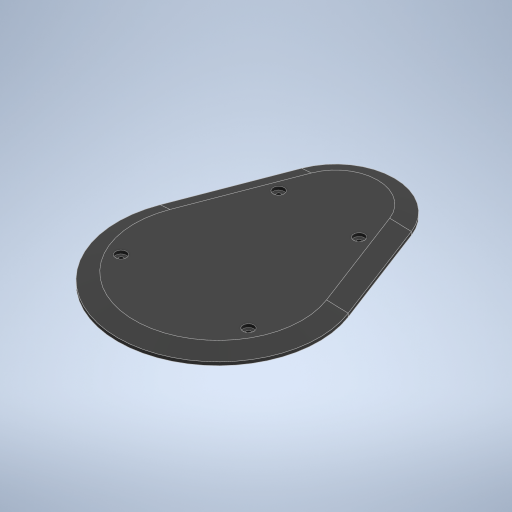
# Autodesk Inventor part: Arm_1_Cover
Saved by Autodesk Inventor 2023 (Build 270158000, 158)
## iProperties
Created: 2024-07-29
Part Number: Arm_1_Cover
Material: Generic
Document SubType Name: Modeling
Designer: Swoby
Density: 1 g/cm^3
Appearance: Default
Author: Swoby
Autodesk Inventor part; units mm, degrees
ref_plane "YZ Plane" through (0, 0, 0) normal (1, 0, 0) x (0, 1, 0)
ref_plane "XZ Plane" through (0, 0, 0) normal (0, 1, 0) x (-1, 0, 0)
ref_plane "XY Plane" through (0, 0, 0) normal (0, 0, 1) x (1, 0, 0)
sketch "Sketch1" plane through (0, 0, 0) normal (0, 1, 0) x (-1, 0, 0)
  arc A0 (28.0215, -10.7143) -> (-28.0215, -10.7143) centre (0, 0) ccw
  arc A1 (14.9976, -25.9821) -> (-16.3459, -41.25) centre (0, -35) ccw construction
  line L0 (0, 0) -> (0, -35) construction
  line L1 (-28.0215, -10.7143) -> (-16.3459, -41.25)
  line L2 (16.3459, -41.25) -> (28.0215, -10.7143)
  arc A2 (14.9976, -25.9821) -> (28.0215, -10.7143) centre (0, 0) ccw construction
  arc A3 (16.3459, -41.25) -> (14.9976, -25.9821) centre (0, -35) ccw construction
  arc A4 (-16.3459, -41.25) -> (16.3459, -41.25) centre (0, -35) ccw
  arc A5 (-28.0215, -10.7143) -> (14.9976, -25.9821) centre (0, 0) ccw construction
  dimension "d0" = 60
  dimension "d1" = 35
  dimension "d2" = 35
  constraints: 12 point on circle, 8 tangent, 6 centre point, 6 end point, 1 coincident, 1 vertical
  measures "d0" diameter of A0
  measures "d1" diameter of A1
  measures "d2" distance of L0.start L0.end
extrude "Extrusion1" add sketch "Sketch1" along normal blind 3
chamfer "Chamfer1" distance 5 distance2 2 4 edges at (0, 3, 30) (22.1837, 3, -25.9821) (0, 3, -52.5) (-22.1837, 3, -25.9821) measured on face at (1.8074, 3, 7.3223)
sketch "Sketch2" plane through (0, 3, 0) normal (0, 1, 0) x (1, 0, 0)
  line L0 (-19, -10) -> (19, -10) construction
  line L1 (19, -10) -> (12, 30) construction
  line L2 (12, 30) -> (-12, 30) construction
  line L3 (-12, 30) -> (-19, -10) construction
  circle A0 centre (-19, -10) radius 0.65
  circle A1 centre (19, -10) radius 0.65
  circle A2 centre (-12, 30) radius 0.65
  circle A3 centre (12, 30) radius 0.65
  point P0 (0, 0)
  dimension "d8" = 10
  dimension "d9" = 30
  dimension "d10" = 19
  dimension "d11" = 19
  dimension "d12" = 12
  dimension "d13" = 12
  dimension "d14" = 1.3
  dimension "d15" = 1.3
  dimension "d16" = 1.3
  dimension "d17" = 1.3
  constraints: 8 end point, 4 centre point, 4 coincident, 1 horizontal, 1 parallel
  measures "d8" distance from line of point (0, 0) L0
  measures "d9" distance from line of L2 point (0, 0)
  measures "d10" horizontal distance of point (0, 0) L0.start
  measures "d11" horizontal distance of L0.end point (0, 0)
  measures "d12" horizontal distance of L2.end point (0, 0)
  measures "d13" horizontal distance of L1.end point (0, 0)
  measures "d14" diameter of A1
  measures "d15" diameter of A2
  measures "d16" diameter of A3
  measures "d17" diameter of A0
extrude "Extrusion2" cut sketch "Sketch2" against normal through all
sketch "Sketch3" plane through (0, 3, 0) normal (0, 1, 0) x (1, 0, 0)
  circle A0 centre (19, -10) radius 0.65 projected
  circle A1 centre (-19, -10) radius 0.65 projected
  arc A2 (-23.3512, 8.9286) -> (23.3512, 8.9286) centre (0, 0) ccw projected
  line L0 (11.6756, 39.4643) -> (23.3512, 8.9286) projected
  arc A3 (11.6756, 39.4643) -> (-11.6756, 39.4643) centre (0, 35) ccw projected
  line L1 (-23.3512, 8.9286) -> (-11.6756, 39.4643) projected
  circle A4 centre (-19, -10) radius 1.65
  circle A5 centre (19, -10) radius 1.65
  circle A6 centre (12, 30) radius 1.65
  circle A7 centre (-12, 30) radius 1.65
  circle A8 centre (-12, 30) radius 0.65 projected
  circle A9 centre (12, 30) radius 0.65 projected
  dimension "d20" = 3.3
  dimension "d21" = 3.3
  dimension "d22" = 3.3
  dimension "d23" = 3.3
  constraints: 4 centre point, 4 coincident
  measures "d20" diameter of A4
  measures "d21" diameter of A5
  measures "d22" diameter of A6
  measures "d23" diameter of A7
extrude "Extrusion3" cut sketch "Sketch3" against normal blind 1 contours A0 | A1 | A4 | A5 | A6 | A7 | A8 | A9
equation "\"d11\" = d10"
equation "\"d13\" = d12"
equation "\"d21\" = d20"
equation "\"d22\" = d20"
equation "\"d23\" = d20"
body "Solid1"
